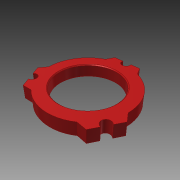
# Autodesk Inventor part: filament_guide_element
Saved by Autodesk Inventor 2014 (Build 180170000, 170)
## iProperties
Created: 2013-12-11
Part Number: filament_guide_element
Material: ABS Plastic
Document SubType Name: Modeling
Designer: buben
Density: 1.06 g/cm^3
Appearance: Light Red
Author: buben
Autodesk Inventor part; units mm, degrees
ref_plane "YZ Plane" through (0, 0, 0) normal (1, 0, 0) x (0, 1, 0)
ref_plane "XZ Plane" through (0, 0, 0) normal (0, 1, 0) x (-1, 0, 0)
ref_plane "XY Plane" through (0, 0, 0) normal (0, 0, 1) x (1, 0, 0)
sketch "Sketch1" plane through (0, 0, 0) normal (0, 0, 1) x (1, 0, 0)
  circle A0 centre (0, 0) radius 10
  arc A1 (-1.4142, 15.5) -> (1.4142, 15.5) centre (0, 15) ccw
  line L0 (1.4142, 15.5) -> (4.4142, 15.5)
  line L1 (-1.4142, 15.5) -> (-4.4142, 15.5)
  line L2 (-4.4142, 15.5) -> (-5.6974, 12.7883)
  line L3 (4.4142, 15.5) -> (5.6974, 12.7883)
  arc A2 (-12.7163, -8.9747) -> (-14.1305, -6.5253) centre (-12.9904, -7.5) ccw
  line L4 (-14.1305, -6.5253) -> (-15.6305, -3.9272)
  line L5 (-12.7163, -8.9747) -> (-11.2163, -11.5728)
  line L6 (-11.2163, -11.5728) -> (-8.2263, -11.3282)
  line L7 (-15.6305, -3.9272) -> (-13.9237, -1.4601)
  arc A3 (14.1305, -6.5253) -> (12.7163, -8.9747) centre (12.9904, -7.5) ccw
  line L8 (12.7163, -8.9747) -> (11.2163, -11.5728)
  line L9 (14.1305, -6.5253) -> (15.6305, -3.9272)
  line L10 (15.6305, -3.9272) -> (13.9237, -1.4601)
  line L11 (11.2163, -11.5728) -> (8.2263, -11.3282)
  arc A4 (-5.6974, 12.7883) -> (-13.9237, -1.4601) centre (0, 0) ccw
  arc A5 (-8.2263, -11.3282) -> (8.2263, -11.3282) centre (0, 0) ccw
  arc A6 (13.9237, -1.4601) -> (5.6974, 12.7883) centre (0, 0) ccw
  dimension "d0" = 20
  dimension "d1" = 3
  dimension "d3" = 15
  dimension "d4" = 3
  dimension "d5" = 0.5
  dimension "d6" = 3
  dimension "d9" = 360
  dimension "d11" = 14
  constraints: 24 end point, 12 point on circle, 7 centre point, 2 coincident, 2 equal length, 1 collinear, 1 horizontal, 1 horizontal alignment, 1 vertical alignment, 37 other
  measures "d0" diameter of A0
  measures "d1" diameter of A1
  measures "d3" distance of point (0, 0) A1.centre
  measures "d4" distance of L1.start L1.end
  measures "d5" distance from line of L1 A1.centre
  measures "d6" distance of L2.end L1.end
  measures "d11" radius of A4
extrude "Extrusion1" add sketch "Sketch1" along normal blind 4
chamfer "Chamfer1" distance 0.3 angle 45 2 edges at (-10, 0, 0) (-10, 0, 4)
body "Solid1"
